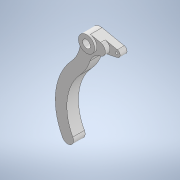
# Autodesk Inventor part: claw-w
Saved by Autodesk Inventor 2020 (Build 240168000, 168)
## iProperties
Created: 2020-11-06
Part Number: claw-w
Material: Generic
Document SubType Name: Modeling
Designer: alnwlsn
Density: 1 g/cm^3
Appearance: Default
Author: alnwlsn
Autodesk Inventor part; units mm, degrees
ref_plane "YZ Plane" through (0, 0, 0) normal (1, 0, 0) x (0, 1, 0)
ref_plane "XZ Plane" through (0, 0, 0) normal (0, 1, 0) x (-1, 0, 0)
ref_plane "XY Plane" through (0, 0, 0) normal (0, 0, 1) x (1, 0, 0)
sketch "Sketch1" plane through (0, 0, 0) normal (0, 0, 1) x (1, 0, 0)
  circle A0 centre (0, 0) radius 2.5
  circle A1 centre (0, 0) radius 3.5
  line L0 (0, 0) -> (10, 0) construction
  circle A2 centre (10, 0) radius 1.5
  circle A3 centre (10, 0) radius 0.5
  line L1 (0.7, 3.4293) -> (10.3, 1.4697)
  line L2 (0.7, -3.4293) -> (10.3, -1.4697)
  dimension "d0" = 5
  dimension "d1" = 7
  dimension "d2" = 3
  dimension "d3" = 1
  dimension "d4" = 10
  constraints: 6 end point, 4 centre point, 4 coincident, 4 point on circle, 4 tangent, 1 horizontal
  measures "d0" diameter of A0
  measures "d1" diameter of A1
  measures "d2" diameter of A2
  measures "d3" diameter of A3
  measures "d4" distance of L0.start L0.end
extrude "Extrusion1" add sketch "Sketch1" along normal blind 3
sketch "Sketch2" plane through (0, 0, 3) normal (0, 0, 1) x (1, 0, 0)
  line L0 (0.7, -3.4293) -> (10.3, -1.4697) projected
  arc A0 (10.3, -1.4697) -> (10.3, 1.4697) centre (10, 0) ccw projected
  line L1 (10.3, 1.4697) -> (0.7, 3.4293) projected
  arc A1 (0.7, 3.4293) -> (0.7, -3.4293) centre (0, 0) ccw projected
  circle A2 centre (10, 0) radius 0.5 projected
  circle A3 centre (0, 0) radius 2.5 projected
  arc A4 (0.7, 3.4293) -> (0.7, -3.4293) centre (0, 0) ccw projected
  circle A5 centre (0, 0) radius 3.5
  point P0 (0.7, -3.4293)
  constraints: 1 coincident, 3 other
extrude "Extrusion2" add sketch "Sketch2" along normal blind 3 contours A1 A5
sketch "Sketch3" plane through (0, 0, 0) normal (0, 0, -1) x (-1, 0, 0)
  line L0 (0, 0) -> (13.4825, -19.2549) construction
  circle A0 centre (-10, 0) radius 0.5 projected
  line L1 (0, 0) -> (-10, 0) construction
  line L2 (0, 0) -> (-9.8298, -6.8829) construction
  circle A1 centre (0, 0) radius 12 construction
  line L3 (-9.8298, -6.8829) -> (6.5648, -30.2969) construction
  circle A2 centre (6.5648, -30.2969) radius 21 construction
  line L4 (0, 0) -> (-12, 0) construction
  line L5 (-12, 0) -> (-12, -49.2406) construction
  circle A3 centre (0, 0) radius 31 construction
  circle A4 centre (-12, -28.5832) radius 21 construction
  arc A5 (11.3096, -41.1892) -> (7.4726, -10.6092) centre (-12, -28.5832) ccw
  arc A6 (-10.3, 1.4697) -> (-10.3, -1.4697) centre (-10, 0) ccw projected
  line L6 (-0.7, -3.4293) -> (-10.3, -1.4697) projected
  arc A7 (-0.7, -3.4293) -> (-0.7, 3.4293) centre (0, 0) ccw projected
  line L7 (-10.3, 1.4697) -> (-0.7, 3.4293) projected
  circle A8 centre (-10, 0) radius 0.5 projected
  circle A9 centre (0, 0) radius 2.5 projected
  arc A10 (3.499, -0.0823) -> (7.4726, -10.6092) centre (18.4949, -0.4352) ccw
  arc A11 (6.9116, -38.8108) -> (3.7986, -14.0005) centre (-12, -28.5832) ccw
  arc A12 (-0.5385, -6.5777) -> (3.7986, -14.0005) centre (18.4949, -0.4352) ccw
  arc A13 (-0.5385, -6.5777) -> (-5.0485, -2.5416) centre (-6.2485, -8.4204) ccw
  line L8 (-10.3, 1.4697) -> (-0.7, 3.4293) projected
  arc A14 (-5.0485, 2.5416) -> (-5.0485, -2.5416) centre (-4.5297, 0) ccw
  line L9 (-0.7, -3.4293) -> (-10.3, -1.4697) projected
  line L10 (-10.3, 1.4697) -> (-0.7, 3.4293) projected
  arc A15 (6.9116, -38.8108) -> (11.3096, -41.1892) centre (9.1106, -40) ccw
  dimension "d10" = 24
  dimension "d9" = 125
  dimension "d11" = 42
  dimension "d12" = 12
  dimension "d13" = 62
  dimension "d14" = 42
  dimension "d17" = 15
  dimension "d18" = 26.5
  dimension "d19" = 5
  dimension "d20" = 5
  dimension "d21" = 6
  dimension "d22" = 40
  constraints: 17 point on circle, 12 end point, 10 centre point, 8 tangent, 4 coincident, 3 perpendicular, 3 point on line, 2 horizontal, 1 concentric, 3 other
  measures "d9" angle of L1 L0
  measures "d11" diameter of A2
  measures "d12" distance of L4.start L4.end
  measures "d13" diameter of A3
  measures "d14" diameter of A4
  measures "d17" radius of A10
  measures "d18" radius of A5
  measures "d19" radial gap between concentric circles of A5 A11
  measures "d20" radial gap between concentric circles of A12 A10
  measures "d21" radius of A13
  measures "d22" vertical distance of A3.centre A15.centre
extrude "Extrusion3" add sketch "Sketch3" against normal blind 5 contours A15 A11 A12 A13 L6 A7 A10 A5 | A7 L6 A14 L7
equation "\"d20\" = d19"
body "Solid1"
